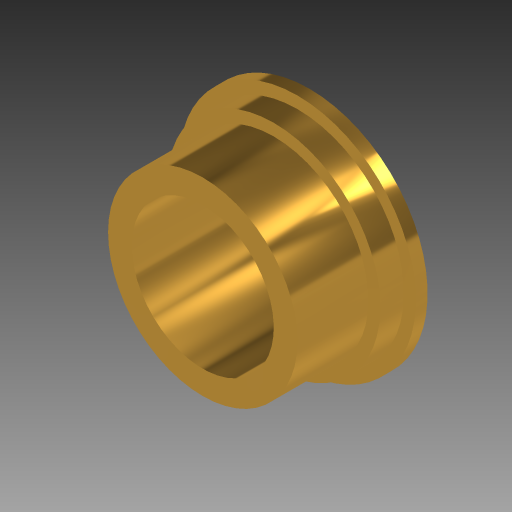
# Autodesk Inventor part: REV MAXSpline Step Bushing
Saved by Autodesk Inventor 2023 (Build 270158000, 158)
## iProperties
Created: 2022-12-26
Part Number: REV MAXSpline Step Bushing
Material: Bronze, Cast
Document SubType Name: Modeling
Designer: Max Boord
Mass: 35.898 g
Surface Area: 30.7191 cm^2
Volume: 4.04713 cm^3
Density: 8.87 g/cm^3
Appearance: Brass - Polished
Author: Max Boord
Autodesk Inventor part; units mm, degrees
ref_plane "YZ Plane" through (0, 0, 0) normal (1, 0, 0) x (0, 1, 0)
ref_plane "XZ Plane" through (0, 0, 0) normal (0, 1, 0) x (-1, 0, 0)
ref_plane "XY Plane" through (0, 0, 0) normal (0, 0, 1) x (1, 0, 0)
sketch "Sketch1" plane through (0, 0, 0) normal (1, 0, 0) x (0, 1, 0)
  line L0 (0, 0) -> (0, 30.2976)
  line L1 (12.7, 9.525) -> (12.7, 0)
  line L2 (12.7, 0) -> (14.2875, 0)
  line L3 (14.2875, 0) -> (14.2875, -3.175)
  line L4 (14.2875, -3.175) -> (15.875, -3.175)
  line L5 (15.875, -3.175) -> (15.875, -4.7625)
  line L6 (15.875, -4.7625) -> (9.525, -4.7625)
  line L7 (9.525, -4.7625) -> (9.525, 9.525)
  line L8 (9.525, 9.525) -> (12.7, 9.525)
  dimension "d0" = 19.05
  dimension "d1" = 1.5875
  dimension "d2" = 3.175
  dimension "d3" = 14.2875
  dimension "d4" = 31.75
  dimension "d5" = 25.4
  dimension "d6" = 28.575
  constraints: 18 end point, 7 perpendicular, 2 vertical, 1 horizontal alignment
  measures "d0" diameter of L7 L0
  measures "d1" distance of L4.end L5.end
  measures "d2" distance of L2.end L3.end
  measures "d3" distance between parallel lines of L6 L8
  measures "d4" diameter of L5 L0
  measures "d5" diameter of L1 L0
  measures "d6" diameter of L3 L0
revolve "Revolution1" add sketch "Sketch1" angle 360 about axis through (0, 0, 0) along (0, 0, 1)
body "Solid1"
